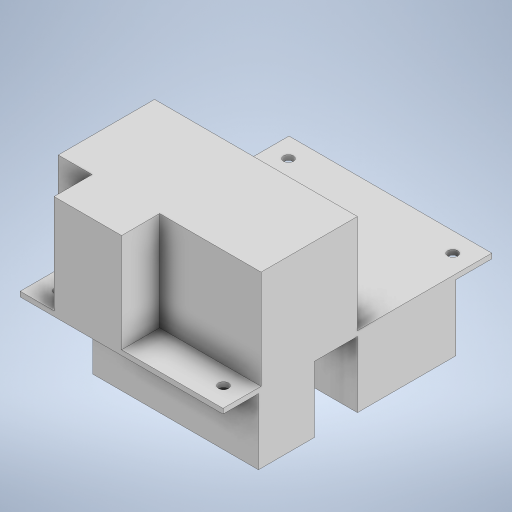
# Autodesk Inventor part: Platine
Saved by Autodesk Inventor 2023 (Build 270158000, 158)
## iProperties
Created: 2022-04-19
Part Number: Platine
Material: Generic
Document SubType Name: Modeling
Designer: benni
Density: 1 g/cm^3
Appearance: Default
Author: benni
Autodesk Inventor part; units mm, degrees
ref_plane "YZ Plane" through (0, 0, 0) normal (1, 0, 0) x (0, 1, 0)
ref_plane "XZ Plane" through (0, 0, 0) normal (0, 1, 0) x (-1, 0, 0)
ref_plane "XY Plane" through (0, 0, 0) normal (0, 0, 1) x (1, 0, 0)
sketch "Sketch1" plane through (0, 0, 0) normal (0, 1, 0) x (-1, 0, 0)
  line L0 (0, 0) -> (61.5, 0)
  line L1 (61.5, 0) -> (61.5, -81.5)
  line L2 (61.5, -81.5) -> (0, -81.5)
  line L3 (0, -81.5) -> (0, 0)
  line L4 (61.5, -40.75) -> (0, -40.75)
  line L5 (30.75, 0) -> (30.75, -81.5)
  line L6 (30.75, -81.5) -> (30.75, 0)
  circle A0 centre (55.65, -6) radius 1.5
  circle A1 centre (5.85, -6) radius 1.5
  circle A2 centre (55.65, -75.5) radius 1.5
  circle A3 centre (5.85, -75.5) radius 1.5
  dimension "d0" = 61.5
  dimension "d1" = 81.5
  dimension "d2" = 69.5
  dimension "d3" = 49.8
  dimension "d4" = 3
  constraints: 14 end point, 10 symmetric about line, 4 centre point, 4 midpoint, 2 coincident, 2 parallel, 1 horizontal, 1 perpendicular, 3 other
  measures "d0" distance of L1.end L2.end
  measures "d1" distance of L0.end L1.end
  measures "d2" diameter of point (55.65, -6) L4
  measures "d3" diameter of point (55.65, -6) L5
  measures "d4" diameter of A0
extrude "Extrusion1" add sketch "Sketch1" along normal blind 1.5
sketch "Sketch2" plane through (0, 1.5, 0) normal (0, 1, 0) x (1, 0, 0)
  line L0 (-61.5, 81.5) -> (-61.5, 0) projected
  line L1 (-61.5, 40.75) -> (0, 40.75)
  line L2 (0, 40.75) -> (0, 11.5412)
  line L3 (0, 11.5412) -> (-61.5, 11.5412)
  line L4 (-61.5, 11.5412) -> (-61.5, 40.75)
  line L5 (-61.5, 0) -> (0, 0) projected
  line L6 (-29.2541, 11.5412) -> (-51.2255, 11.5412)
  line L7 (-61.5, 68.5681) -> (-61.5, 63.2604)
  line L8 (-51.2255, 11.5412) -> (-30.75, 11.5412)
  line L9 (-30.75, 11.5412) -> (-30.75, 0)
  line L10 (-30.75, 0) -> (-51.2255, 0)
  line L11 (-51.2255, 0) -> (-51.2255, 11.5412)
  point P0 (0, 68.5681)
  constraints: 20 end point, 4 parallel, 3 point on line, 2 horizontal, 2 midpoint, 2 perpendicular
extrude "Extrusion2" add sketch "Sketch2" along normal blind 30 contours L1 L2 L3 L0 | L3 L9 L5 L11
sketch "Sketch3" plane through (0, 0, 0) normal (0, -1, 0) x (1, 0, 0)
  line L0 (-61.5, -81.5) -> (-61.5, 0) projected
  line L1 (-61.5, -40.75) -> (0, -40.75) projected
  line L2 (-61.5, -70.6132) -> (0, -70.6132)
  line L3 (0, -70.6132) -> (0, -40.75)
  line L4 (0, -40.75) -> (-61.5, -40.75)
  line L5 (-61.5, -40.75) -> (-61.5, -70.6132)
  line L6 (0, 0) -> (0, -81.5) projected
  line L7 (-50.2544, -10.7457) -> (0, -10.7457)
  line L8 (0, -10.7457) -> (0, -27.6996)
  line L9 (0, -27.6996) -> (-50.2544, -27.6996)
  line L10 (-50.2544, -27.6996) -> (-50.2544, -10.7457)
  constraints: 16 end point, 4 parallel, 2 horizontal, 2 perpendicular, 2 point on line
extrude "Extrusion3" add sketch "Sketch3" along normal blind 20
body "Solid1"
